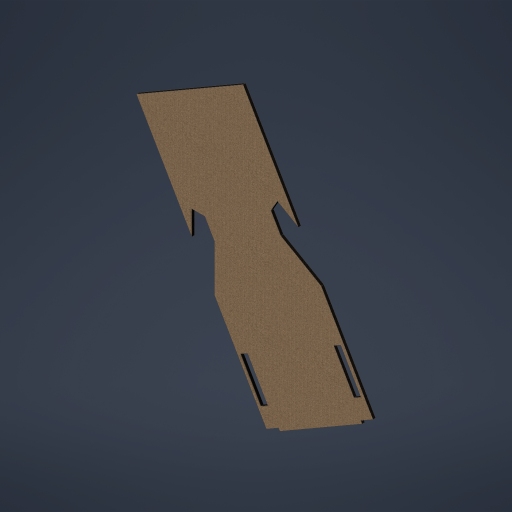
# Autodesk Inventor part: Cover_Back
Saved by Autodesk Inventor 2024.1 (Build 281209000, 209)
## iProperties
Created: 2023-08-06
Part Number: Cover_Back
Material: MDF Medium Density Fiberboard
Document SubType Name: Modeling
Designer: jaege
Density: 0.8 g/cm^3
Appearance: Cardboard - Corrugated
Author: jaege
Autodesk Inventor part; units mm, degrees
ref_plane "YZ Plane" through (0, 0, 0) normal (1, 0, 0) x (0, 1, 0)
ref_plane "XZ Plane" through (0, 0, 0) normal (0, 1, 0) x (-1, 0, 0)
ref_plane "XY Plane" through (0, 0, 0) normal (0, 0, 1) x (1, 0, 0)
sketch "Sketch1" plane through (0, 0, 0) normal (0, 0, 1) x (1, 0, 0)
  line L0 (-90.0173, 111.9145) -> (73.6615, 206.4145)
  line L1 (73.6615, 206.4145) -> (275.1615, -142.5937)
  line L2 (275.1615, -142.5937) -> (130.1022, -226.3437)
  line L3 (111.4827, -237.0937) -> (109.4827, -233.6296) construction
  line L4 (89.6429, -179.2661) -> (74.6429, -153.2854) construction
  line L5 (74.6429, -153.2854) -> (65.7952, -137.9607) construction
  line L6 (69.2593, -135.9607) -> (65.7952, -137.9607) construction
  line L7 (69.2593, -135.9607) -> (78.1071, -151.2854) construction
  line L8 (78.1071, -151.2854) -> (93.1071, -177.2661) construction
  line L9 (93.1071, -177.2661) -> (89.6429, -179.2661) construction
  line L10 (74.6429, -153.2854) -> (78.1071, -151.2854) construction
  line L11 (-4, -30) -> (-4, 0) construction
  line L12 (-4, 0) -> (-4, 17.6954) construction
  line L13 (0, 17.6954) -> (-4, 17.6954) construction
  line L14 (0, 17.6954) -> (0, 0) construction
  line L15 (0, 0) -> (0, -30) construction
  line L16 (0, -30) -> (-4, -30) construction
  line L17 (-4, 0) -> (0, 0) construction
  line L18 (151.5544, 57.5) -> (125.5737, 72.5) construction
  line L19 (125.5737, 72.5) -> (110.249, 81.3477) construction
  line L20 (112.249, 84.8118) -> (110.249, 81.3477) construction
  line L21 (112.249, 84.8118) -> (127.5737, 75.9641) construction
  line L22 (127.5737, 75.9641) -> (153.5544, 60.9641) construction
  line L23 (153.5544, 60.9641) -> (151.5544, 57.5) construction
  line L24 (125.5737, 72.5) -> (127.5737, 75.9641) construction
  line L25 (232.5371, -96.7661) -> (217.5371, -70.7854) construction
  line L26 (217.5371, -70.7854) -> (208.6894, -55.4607) construction
  line L27 (212.1535, -53.4607) -> (208.6894, -55.4607) construction
  line L28 (212.1535, -53.4607) -> (221.0012, -68.7854) construction
  line L29 (221.0012, -68.7854) -> (236.0012, -94.7661) construction
  line L30 (236.0012, -94.7661) -> (232.5371, -96.7661) construction
  line L31 (217.5371, -70.7854) -> (221.0012, -68.7854) construction
  line L32 (142.8942, 62.5) -> (129.9038, 70) construction
  line L33 (129.9038, 70) -> (187.774, -30.2341) construction
  line L34 (187.774, -30.2341) -> (57.8702, -105.2341) construction
  line L35 (57.8702, -105.2341) -> (0, -5) construction
  line L36 (0, -5) -> (0, -20) construction
  line L37 (0, -20) -> (-4, -20) construction
  line L38 (-4, -20) -> (-4, 1.9282) construction
  line L39 (-4, 1.9282) -> (-65.6298, 108.6742) construction
  line L40 (-65.6298, 108.6742) -> (64.274, 183.6742) construction
  line L41 (64.274, 183.6742) -> (125.9038, 76.9282) construction
  line L42 (125.9038, 76.9282) -> (144.8942, 65.9641) construction
  line L43 (144.8942, 65.9641) -> (142.8942, 62.5) construction
  circle A0 centre (93.125, -181.2972) radius 1.5 construction
  circle A1 centre (-2, -33.5) radius 1.5 construction
  circle A2 centre (236.0192, -98.7972) radius 1.5 construction
  line L44 (57.1429, -122.9745) -> (60.6071, -120.9745) construction
  line L45 (60.6071, -120.9745) -> (88.1071, -168.6059) construction
  line L46 (88.1071, -168.6059) -> (84.6429, -170.6059) construction
  line L47 (84.6429, -170.6059) -> (57.1429, -122.9745) construction
  line L48 (200.0371, -40.4745) -> (203.5012, -38.4745) construction
  line L49 (203.5012, -38.4745) -> (231.0012, -86.1059) construction
  line L50 (231.0012, -86.1059) -> (227.5371, -88.1059) construction
  line L51 (227.5371, -88.1059) -> (200.0371, -40.4745) construction
  circle A3 centre (155.5855, 57.4821) radius 1.5 construction
  line L52 (240.274, -121.1668) -> (261.274, -157.5398) construction
  line L53 (272.0993, -151.2898) -> (261.274, -157.5398) construction
  line L54 (268.0993, -144.3616) -> (272.0993, -151.2898) construction
  line L55 (268.0993, -144.3616) -> (299.7092, -126.1116) construction
  line L56 (299.7092, -126.1116) -> (281.7092, -94.9347) construction
  line L57 (281.7092, -94.9347) -> (277.5523, -97.3347) construction
  line L58 (277.5523, -97.3347) -> (278.1523, -98.374) construction
  line L59 (278.1523, -98.374) -> (276.0739, -99.574) construction
  line L60 (276.0739, -99.574) -> (275.4739, -98.5347) construction
  line L61 (275.4739, -98.5347) -> (271.3169, -100.9347) construction
  line L62 (271.3169, -100.9347) -> (269.8169, -98.3367) construction
  line L63 (269.8169, -98.3367) -> (273.9739, -95.9367) construction
  line L64 (273.9739, -95.9367) -> (273.3739, -94.8974) construction
  line L65 (273.3739, -94.8974) -> (275.4523, -93.6974) construction
  line L66 (275.4523, -93.6974) -> (276.0523, -94.7367) construction
  line L67 (276.0523, -94.7367) -> (280.2092, -92.3367) construction
  line L68 (280.2092, -92.3367) -> (262.2092, -61.1597) construction
  line L69 (262.2092, -61.1597) -> (265.6733, -59.1597) construction
  line L70 (265.6733, -59.1597) -> (228.1733, 5.7922) construction
  line L71 (228.1733, 5.7922) -> (224.7092, 3.7922) construction
  line L72 (224.7092, 3.7922) -> (206.7092, 34.9691) construction
  line L73 (206.7092, 34.9691) -> (202.5523, 32.5691) construction
  line L74 (202.5523, 32.5691) -> (203.1523, 31.5299) construction
  line L75 (203.1523, 31.5299) -> (201.0739, 30.3299) construction
  line L76 (201.0739, 30.3299) -> (200.4739, 31.3691) construction
  line L77 (200.4739, 31.3691) -> (196.3169, 28.9691) construction
  line L78 (196.3169, 28.9691) -> (194.8169, 31.5672) construction
  line L79 (194.8169, 31.5672) -> (198.9739, 33.9672) construction
  line L80 (198.9739, 33.9672) -> (198.3739, 35.0064) construction
  line L81 (198.3739, 35.0064) -> (200.4523, 36.2064) construction
  line L82 (200.4523, 36.2064) -> (201.0523, 35.1672) construction
  line L83 (201.0523, 35.1672) -> (205.2092, 37.5672) construction
  line L84 (205.2092, 37.5672) -> (187.2092, 68.7441) construction
  line L85 (187.2092, 68.7441) -> (190.6733, 70.7441) construction
  line L86 (190.6733, 70.7441) -> (153.1733, 135.696) construction
  line L87 (153.1733, 135.696) -> (149.7092, 133.696) construction
  line L88 (149.7092, 133.696) -> (131.7092, 164.8729) construction
  line L89 (131.7092, 164.8729) -> (127.5523, 162.4729) construction
  line L90 (127.5523, 162.4729) -> (128.1523, 161.4337) construction
  line L91 (128.1523, 161.4337) -> (126.0739, 160.2337) construction
  line L92 (126.0739, 160.2337) -> (125.4739, 161.2729) construction
  line L93 (125.4739, 161.2729) -> (121.3169, 158.8729) construction
  line L94 (121.3169, 158.8729) -> (119.8169, 161.471) construction
  line L95 (119.8169, 161.471) -> (123.9739, 163.871) construction
  line L96 (123.9739, 163.871) -> (123.3739, 164.9102) construction
  line L97 (123.3739, 164.9102) -> (125.4523, 166.1102) construction
  line L98 (125.4523, 166.1102) -> (126.0523, 165.071) construction
  line L99 (126.0523, 165.071) -> (130.2092, 167.471) construction
  line L100 (130.2092, 167.471) -> (112.2092, 198.6479) construction
  line L101 (112.2092, 198.6479) -> (115.6733, 200.6479) construction
  line L102 (115.6733, 200.6479) -> (78.1733, 265.5998) construction
  line L103 (78.1733, 265.5998) -> (57.3887, 253.5998) construction
  line L104 (57.3887, 253.5998) -> (94.8887, 188.6479) construction
  line L105 (91.4246, 186.6479) -> (94.8887, 188.6479) construction
  line L106 (53.9246, 251.5998) -> (91.4246, 186.6479) construction
  line L107 (43.0993, 245.3498) -> (53.9246, 251.5998) construction
  line L108 (41.0993, 248.8139) -> (43.0993, 245.3498) construction
  line L109 (10.7884, 231.3139) -> (41.0993, 248.8139) construction
  line L110 (12.7884, 227.8498) -> (10.7884, 231.3139) construction
  line L111 (-1.068, 219.8498) -> (12.7884, 227.8498) construction
  line L112 (1.332, 215.6929) -> (-1.068, 219.8498) construction
  line L113 (2.3713, 216.2929) -> (1.332, 215.6929) construction
  line L114 (3.5713, 214.2144) -> (2.3713, 216.2929) construction
  line L115 (2.532, 213.6144) -> (3.5713, 214.2144) construction
  line L116 (4.932, 209.4575) -> (2.532, 213.6144) construction
  line L117 (2.3339, 207.9575) -> (4.932, 209.4575) construction
  line L118 (-0.0661, 212.1144) -> (2.3339, 207.9575) construction
  line L119 (-1.1053, 211.5144) -> (-0.0661, 212.1144) construction
  line L120 (-2.3053, 213.5929) -> (-1.1053, 211.5144) construction
  line L121 (-1.2661, 214.1929) -> (-2.3053, 213.5929) construction
  line L122 (-3.6661, 218.3498) -> (-1.2661, 214.1929) construction
  line L123 (-17.5225, 210.3498) -> (-3.6661, 218.3498) construction
  line L124 (-19.5225, 213.8139) -> (-17.5225, 210.3498) construction
  line L125 (-49.8333, 196.3139) -> (-19.5225, 213.8139) construction
  line L126 (-47.8333, 192.8498) -> (-49.8333, 196.3139) construction
  line L127 (-61.6898, 184.8498) -> (-47.8333, 192.8498) construction
  line L128 (-59.2898, 180.6929) -> (-61.6898, 184.8498) construction
  line L129 (-58.2505, 181.2929) -> (-59.2898, 180.6929) construction
  line L130 (-57.0505, 179.2144) -> (-58.2505, 181.2929) construction
  line L131 (-58.0898, 178.6144) -> (-57.0505, 179.2144) construction
  line L132 (-55.6898, 174.4575) -> (-58.0898, 178.6144) construction
  line L133 (-58.2878, 172.9575) -> (-55.6898, 174.4575) construction
  line L134 (-60.6878, 177.1144) -> (-58.2878, 172.9575) construction
  line L135 (-61.7271, 176.5144) -> (-60.6878, 177.1144) construction
  line L136 (-62.9271, 178.5929) -> (-61.7271, 176.5144) construction
  line L137 (-61.8878, 179.1929) -> (-62.9271, 178.5929) construction
  line L138 (-64.2878, 183.3498) -> (-61.8878, 179.1929) construction
  line L139 (-78.1442, 175.3498) -> (-64.2878, 183.3498) construction
  line L140 (-80.1442, 178.8139) -> (-78.1442, 175.3498) construction
  line L141 (-110.4551, 161.3139) -> (-80.1442, 178.8139) construction
  line L142 (-108.4551, 157.8498) -> (-110.4551, 161.3139) construction
  line L143 (-122.7445, 149.5998) -> (-108.4551, 157.8498) construction
  line L144 (-85.2445, 84.6479) -> (-122.7445, 149.5998) construction
  line L145 (-81.7804, 86.6479) -> (-85.2445, 84.6479) construction
  line L146 (-63.7804, 55.471) -> (-81.7804, 86.6479) construction
  line L147 (-63.7804, 55.471) -> (-59.6235, 57.871) construction
  line L148 (-59.6235, 57.871) -> (-60.2235, 58.9102) construction
  line L149 (-60.2235, 58.9102) -> (-58.1451, 60.1102) construction
  line L150 (-58.1451, 60.1102) -> (-57.5451, 59.071) construction
  line L151 (-57.5451, 59.071) -> (-53.3881, 61.471) construction
  line L152 (-53.3881, 61.471) -> (-51.8881, 58.8729) construction
  line L153 (-51.8881, 58.8729) -> (-56.0451, 56.4729) construction
  line L154 (-56.0451, 56.4729) -> (-55.4451, 55.4337) construction
  line L155 (-55.4451, 55.4337) -> (-57.5235, 54.2337) construction
  line L156 (-57.5235, 54.2337) -> (-58.1235, 55.2729) construction
  line L157 (-58.1235, 55.2729) -> (-62.2804, 52.8729) construction
  line L158 (-44.2804, 21.696) -> (-62.2804, 52.8729) construction
  line L159 (-47.7445, 19.696) -> (-44.2804, 21.696) construction
  line L160 (-10.2445, -45.2559) -> (-47.7445, 19.696) construction
  line L161 (-6.7804, -43.2559) -> (-10.2445, -45.2559) construction
  line L162 (11.2196, -74.4328) -> (-6.7804, -43.2559) construction
  line L163 (11.2196, -74.4328) -> (15.3765, -72.0328) construction
  line L164 (15.3765, -72.0328) -> (14.7765, -70.9936) construction
  line L165 (14.7765, -70.9936) -> (16.8549, -69.7936) construction
  line L166 (16.8549, -69.7936) -> (17.4549, -70.8328) construction
  line L167 (17.4549, -70.8328) -> (21.6119, -68.4328) construction
  line L168 (21.6119, -68.4328) -> (23.1119, -71.0309) construction
  line L169 (23.1119, -71.0309) -> (18.9549, -73.4309) construction
  line L170 (18.9549, -73.4309) -> (19.5549, -74.4701) construction
  line L171 (19.5549, -74.4701) -> (17.4765, -75.6701) construction
  line L172 (17.4765, -75.6701) -> (16.8765, -74.6309) construction
  line L173 (16.8765, -74.6309) -> (12.7196, -77.0309) construction
  line L174 (30.7196, -108.2078) -> (12.7196, -77.0309) construction
  line L175 (27.2555, -110.2078) -> (30.7196, -108.2078) construction
  line L176 (64.7555, -175.1597) -> (27.2555, -110.2078) construction
  line L177 (68.2196, -173.1597) -> (64.7555, -175.1597) construction
  line L178 (86.2196, -204.3367) -> (68.2196, -173.1597) construction
  line L179 (86.2196, -204.3367) -> (90.3765, -201.9367) construction
  line L180 (90.3765, -201.9367) -> (89.7765, -200.8974) construction
  line L181 (89.7765, -200.8974) -> (91.8549, -199.6974) construction
  line L182 (91.8549, -199.6974) -> (92.4549, -200.7367) construction
  line L183 (92.4549, -200.7367) -> (96.6119, -198.3367) construction
  line L184 (96.6119, -198.3367) -> (98.1119, -200.9347) construction
  line L185 (98.1119, -200.9347) -> (93.9549, -203.3347) construction
  line L186 (93.9549, -203.3347) -> (94.5549, -204.374) construction
  line L187 (94.5549, -204.374) -> (92.4765, -205.574) construction
  line L188 (92.4765, -205.574) -> (91.8765, -204.5347) construction
  line L189 (91.8765, -204.5347) -> (87.7196, -206.9347) construction
  line L190 (105.7196, -238.1116) -> (87.7196, -206.9347) construction
  line L191 (116.5449, -231.8616) -> (105.7196, -238.1116) construction
  line L192 (120.5449, -238.7898) -> (116.5449, -231.8616) construction
  line L193 (131.3702, -232.5398) -> (120.5449, -238.7898) construction
  line L194 (131.3702, -232.5398) -> (110.3702, -196.1668) construction
  line L195 (110.3702, -196.1668) -> (240.274, -121.1668) construction
  line L196 (241.4246, -73.1597) -> (244.8887, -71.1597) construction
  line L197 (203.9246, -8.2078) -> (241.4246, -73.1597) construction
  line L198 (207.3887, -6.2078) -> (203.9246, -8.2078) construction
  line L199 (207.3887, -6.2078) -> (244.8887, -71.1597) construction
  line L200 (166.4246, 56.7441) -> (169.8887, 58.7441) construction
  line L201 (128.9246, 121.696) -> (166.4246, 56.7441) construction
  line L202 (132.3887, 123.696) -> (128.9246, 121.696) construction
  line L203 (132.3887, 123.696) -> (169.8887, 58.7441) construction
  circle A4 centre (245.1913, -27.6838) radius 1.5 construction
  circle A5 centre (170.1913, 102.22) radius 1.5 construction
  circle A6 centre (95.1913, 232.1238) radius 1.5 construction
  circle A7 centre (-40.4936, 160.137) radius 1.5 construction
  circle A8 centre (7.1378, 187.637) radius 1.5 construction
  circle A9 centre (162.6378, -81.6969) radius 1.5 construction
  circle A10 centre (115.0064, -109.1969) radius 1.5 construction
  circle A11 centre (148.5064, -167.2206) radius 1.5 construction
  circle A12 centre (196.1378, -139.7206) radius 1.5 construction
  line L204 (107.3461, -115.929) -> (77.0353, -133.429) construction
  line L205 (77.0353, -133.429) -> (75.0353, -129.9649) construction
  line L206 (75.0353, -129.9649) -> (105.3461, -112.4649) construction
  line L207 (105.3461, -112.4649) -> (107.3461, -115.929) construction
  line L208 (45.1089, 211.869) -> (47.1089, 208.4049) construction
  line L209 (47.1089, 208.4049) -> (16.798, 190.9049) construction
  line L210 (16.798, 190.9049) -> (14.798, 194.369) construction
  line L211 (14.798, 194.369) -> (45.1089, 211.869) construction
  line L212 (-32.8333, 166.869) -> (-2.5225, 184.369) construction
  line L213 (-2.5225, 184.369) -> (-0.5225, 180.9049) construction
  line L214 (-0.5225, 180.9049) -> (-30.8333, 163.4049) construction
  line L215 (-30.8333, 163.4049) -> (-32.8333, 166.869) construction
  line L216 (140.8461, -173.9527) -> (110.5353, -191.4527) construction
  line L217 (110.5353, -191.4527) -> (108.5353, -187.9886) construction
  line L218 (108.5353, -187.9886) -> (138.8461, -170.4886) construction
  line L219 (138.8461, -170.4886) -> (140.8461, -173.9527) construction
  line L220 (154.9775, -88.429) -> (124.6667, -105.929) construction
  line L221 (124.6667, -105.929) -> (122.6667, -102.4649) construction
  line L222 (122.6667, -102.4649) -> (152.9775, -84.9649) construction
  line L223 (152.9775, -84.9649) -> (154.9775, -88.429) construction
  line L224 (236.1089, -118.9527) -> (205.798, -136.4527) construction
  line L225 (205.798, -136.4527) -> (203.798, -132.9886) construction
  line L226 (203.798, -132.9886) -> (234.1089, -115.4886) construction
  line L227 (234.1089, -115.4886) -> (236.1089, -118.9527) construction
  line L228 (-48.1539, 153.4049) -> (-78.4647, 135.9049) construction
  line L229 (-78.4647, 135.9049) -> (-80.4647, 139.369) construction
  line L230 (-80.4647, 139.369) -> (-50.1539, 156.869) construction
  line L231 (-50.1539, 156.869) -> (-48.1539, 153.4049) construction
  line L232 (186.4775, -142.9886) -> (188.4775, -146.4527) construction
  line L233 (188.4775, -146.4527) -> (158.1667, -163.9527) construction
  line L234 (158.1667, -163.9527) -> (156.1667, -160.4886) construction
  line L235 (156.1667, -160.4886) -> (186.4775, -142.9886) construction
  line L236 (200.6089, -57.4649) -> (202.6089, -60.929) construction
  line L237 (202.6089, -60.929) -> (172.298, -78.429) construction
  line L238 (172.298, -78.429) -> (170.298, -74.9649) construction
  line L239 (170.298, -74.9649) -> (200.6089, -57.4649) construction
  circle A13 centre (-27.2625, -11.78) radius 1.5 construction
  circle A14 centre (47.7375, -141.6838) radius 1.5 construction
  circle A15 centre (186.9067, 25.2681) radius 1.5 construction
  circle A16 centre (111.9067, 155.1719) radius 1.5 construction
  circle A17 centre (261.9067, -104.6357) radius 1.5 construction
  circle A18 centre (-102.2625, 118.1238) radius 1.5 construction
  line L240 (116.5449, -231.8616) -> (268.0993, -144.3616) construction
  line L241 (118.5449, -235.3257) -> (116.5449, -231.8616) construction
  line L242 (118.5449, -235.3257) -> (270.0993, -147.8257) construction
  line L243 (270.0993, -147.8257) -> (268.0993, -144.3616) construction
  line L244 (284.3887, -139.5757) -> (104.2555, -243.5757) construction
  line L245 (104.2555, -243.5757) -> (106.2555, -247.0398) construction
  line L246 (286.3887, -143.0398) -> (106.2555, -247.0398) construction
  line L247 (284.3887, -139.5757) -> (286.3887, -143.0398) construction
  line L248 (-5, 1.7321) -> (29.99, 1.7321) construction
  line L249 (29.99, 1.7321) -> (29.99, -35.3397) construction
  line L250 (29.99, -35.3397) -> (-5, -35.3397) construction
  line L251 (-5, -35.3397) -> (-5, 1.7321)
  line L252 (14.99, 1.7321) -> (29.99, -24.2487)
  line L253 (29.99, -24.2487) -> (29.99, -95.9441)
  line L254 (-5, 1.7321) -> (14.99, 1.7321)
  line L255 (70.1788, -153.5533) -> (80.5712, -147.5533)
  line L256 (80.5712, -147.5533) -> (111.5712, -201.2469)
  line L257 (111.5712, -201.2469) -> (101.1788, -207.2469)
  line L258 (101.1788, -207.2469) -> (70.1788, -153.5533)
  line L259 (111.4827, -237.0937) -> (130.1022, -226.3437) construction
  line L260 (130.1022, -226.3437) -> (128.1022, -222.8796)
  line L261 (128.1022, -222.8796) -> (109.4827, -233.6296)
  line L262 (109.4827, -233.6296) -> (111.4827, -237.0937) construction
  line L263 (109.4827, -233.6296) -> (-90.0173, 111.9145)
  line L264 (130.1022, -226.3437) -> (111.4827, -237.0937) construction
  line L265 (-0.6779, 146.1742) -> (194.3221, -191.5757) construction
  line L266 (158.6788, 59.1603) -> (126.5737, 77.6962)
  line L267 (116.5787, 60.3843) -> (131.5787, 34.4036)
  line L268 (131.5787, 34.4036) -> (193.6688, -1.4441)
  line L269 (126.5737, 77.6962) -> (116.5787, 60.3843)
  line L270 (223.4653, -65.0533) -> (213.073, -71.0533)
  line L271 (213.073, -71.0533) -> (244.073, -124.7469)
  line L272 (244.073, -124.7469) -> (254.4653, -118.7469)
  line L273 (254.4653, -118.7469) -> (223.4653, -65.0533)
  line L274 (256.542, -153.3437) -> (254.542, -149.8796)
  line L275 (254.542, -149.8796) -> (273.1615, -139.1296)
  line L276 (-4, 0) -> (-5, 1.7321) construction
  line L277 (-5, 1.7321) -> (-5, 1.7321) construction
  point P0 (75.375, -150.5533)
  point P1 (193.6688, -1.4441)
  dimension "d0" = 2
  dimension "d1" = 10
  dimension "d2" = 10
  dimension "d3" = 1
  dimension "d5" = 5
  dimension "d7" = 30
  dimension "d8" = 4
  dimension "d9" = 4
  dimension "d12" = 30
  dimension "d13" = 2
  dimension "d14" = 2
  dimension "d17" = 2
  dimension "d18" = 15
  dimension "d19" = 2
  constraints: 124 end point, 19 parallel, 12 symmetric about line, 6 point on line, 5 perpendicular, 4 vertical, 3 horizontal, 3 midpoint, 44 other
  measures "d0" distance between parallel lines of L244 L2
  measures "d1" distance between parallel lines of L3 L47
  measures "d2" distance between parallel lines of L1 L49
  measures "d3" distance between parallel lines of L11 L251
  measures "d5" distance from line of L252 L13.start
  measures "d7" distance of L252.start L252.end
  measures "d8" distance between parallel lines of L47 L258
  measures "d9" distance between parallel lines of L256 L45
  measures "d12" distance between parallel lines of L257 L9
  measures "d13" distance between parallel lines of L240 L261
  measures "d14" distance between parallel lines of L194 L260
  measures "d17" distance of L11.end L276.end
  measures "d18" distance between parallel lines of L40 L0
  measures "d19" distance between parallel lines of L10 L255
extrude "Extrusion1" add sketch "Sketch1" along normal blind 4 contours L0 L1 L266 L269 L267 L268 L275 L274 L2 L260 L261 L263 L253 L252 L254 L251
body "Solid1"
